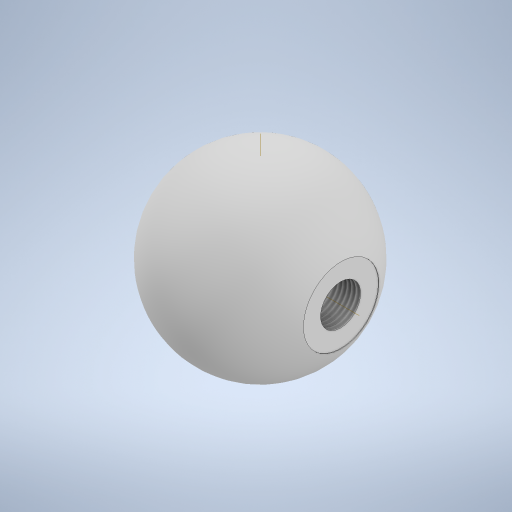
# Autodesk Inventor part: Knob
Saved by Autodesk Inventor 2024 (Build 280153000, 153)
## iProperties
Created: 2023-11-09
Part Number: Knob
Material: Generic
Document SubType Name: Modeling
Designer: Admin
Density: 1 g/cm^3
Appearance: Default
Author: Admin
Autodesk Inventor part; units mm, degrees
ref_plane "XZ Plane" through (0, 0, 0) normal (0, 1, 0) x (-1, 0, 0)
ref_plane "XY Plane" through (0, 0, 0) normal (0, 0, 1) x (1, 0, 0)
sketch "Sketch3" plane through (0, 0, 0) normal (1, 0, 0) x (0, 1, 0)
  arc A0 (0, -20) -> (0, 20) centre (0, 0) ccw
  line L0 (0, 20) -> (0, -20)
  line L1 (0, -28) -> (0, 28) projected
  dimension "d15" = 20
  constraints: 2 end point, 2 point on circle, 1 centre point, 1 coincident, 1 vertical
  measures "d15" radius of A0
revolve "Revolution4" add sketch "Sketch3" angle 360 about axis through (0, 0, -10) along (0, 0, 1)
ref_plane "Work Plane2" through (18, 0, 0) normal (1, 0, 0) x (0, 1, 0)
sketch "Sketch4" plane through (18, 0, 0) normal (1, 0, 0) x (0, 1, 0)
  circle A0 centre (0, 0) radius 8.4531
  circle A1 centre (0, 0) radius 4.5
  dimension "d20" = 9
  constraints: 3 coincident, 2 centre point
  measures "d20" diameter of A1
extrude "Extrusion4" cut sketch "Sketch4" along normal through all contours A0 | A1
hole "Hole1" at (18, 0, 0) direction (-1, 0, 0) diameter 9 depth 10 tip angle 118
thread "Thread1" size "M10x1" class "6H" standard "ANSI Metric M Profile" length 56
body "Solid4"
